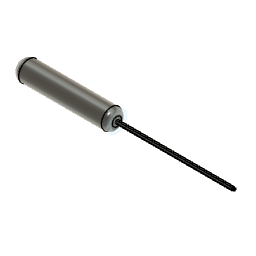
screwdriver v1 (Autodesk Fusion 360 design; units mm, degrees)
Autodesk Fusion 360 part; units mm, degrees
sketch "Sketch1" plane through (0, 0, 0) normal (1, 0, 0) x (0, 1, 0)
  circle A0 centre (0, 80) radius 13.595
  dimension "d2" = 27.19
  measures "d2" diameter of A0
extrude "Extrude1" add sketch "Sketch1" along normal blind 130
sketch "Sketch2" plane through (130, 0, 0) normal (1, 0, 0) x (0, 1, 0)
  circle A0 centre (0, 80) radius 13.595
  line L0 (1.1547, 78) -> (2.3094, 80)
  line L1 (2.3094, 80) -> (1.1547, 82)
  line L2 (1.1547, 82) -> (-1.1547, 82)
  line L3 (-1.1547, 82) -> (-2.3094, 80)
  line L4 (-2.3094, 80) -> (-1.1547, 78)
  line L5 (-1.1547, 78) -> (1.1547, 78)
  point P0 (0, 80)
  dimension "d5" = 2
  constraint coincident P0 A0.centre
  measures "d5" distance of P0 L5
extrude "Extrude2" add sketch "Sketch2" along normal blind 160 contours L0 L1 L2 L3 L4 L5
chamfer "Chamfer1" distance 1 angle 45 6 edges at (290, -1.7321, 81) (290, 0, 82) (290, -1.7321, 79) (290, 0, 78) (290, 1.7321, 79) (290, 1.7321, 81)
sketch "Sketch3" plane through (130, 0, 0) normal (1, 0, 0) x (0, 1, 0)
  line L0 (-1.1547, 78) -> (-2.3094, 80)
  line L1 (-2.3094, 80) -> (-1.1547, 82)
  line L2 (-1.1547, 82) -> (1.1547, 82)
  line L3 (1.1547, 82) -> (2.3094, 80)
  line L4 (2.3094, 80) -> (1.1547, 78)
  line L5 (1.1547, 78) -> (-1.1547, 78)
  circle A0 centre (0, 80) radius 13.595
sketch "Sketch4" plane through (290, 0, 0) normal (1, 0, 0) x (0, 1, 0)
  line L0 (0.5774, 79) -> (1.1547, 80)
  line L1 (1.1547, 80) -> (0.5774, 81)
  line L2 (0.5774, 81) -> (-0.5774, 81)
  line L3 (-0.5774, 81) -> (-1.1547, 80)
  line L4 (-1.1547, 80) -> (-0.5774, 79)
  line L5 (-0.5774, 79) -> (0.5774, 79)
  line L6 (-0.2, 80.1) -> (-0.2, 82.1)
  line L7 (-0.2, 82.1) -> (-2.8, 82.1)
  line L8 (-2.8, 82.1) -> (-2.8, 80.1)
  line L9 (-2.8, 80.1) -> (-0.2, 80.1)
  line L10 (0.2, 80.1) -> (0.2, 82.1)
  line L11 (0.2, 82.1) -> (2.8, 82.1)
  line L12 (2.8, 82.1) -> (2.8, 80.1)
  line L13 (2.8, 80.1) -> (0.2, 80.1)
  line L14 (0.2, 79.8) -> (2.8, 79.8)
  line L15 (2.8, 79.8) -> (2.8, 77.7841)
  line L16 (2.8, 77.7841) -> (0.2, 77.7841)
  line L17 (0.2, 77.7841) -> (0.2, 79.8)
  line L18 (-0.2, 79.8) -> (-0.2, 77.7841)
  line L19 (-0.2, 77.7841) -> (-2.5, 77.5)
  line L20 (-2.5, 77.5) -> (-2.5, 79.8)
  line L21 (-2.5, 79.8) -> (-0.2, 79.8)
  constraint perpendicular L2 L6
  constraint perpendicular L6 L7
  constraint perpendicular L7 L8
  constraint perpendicular L6 L9
  constraint perpendicular L9 L10
  constraint perpendicular L6 L11
  constraint perpendicular L11 L12
  constraint perpendicular L10 L13
  constraint perpendicular L10 L14
  constraint perpendicular L14 L15
  constraint perpendicular L10 L16
  constraint perpendicular L14 L17
  constraint perpendicular L5 L18
  constraint perpendicular L5 L20
  constraint perpendicular L18 L21
extrude "Extrude3" cut sketch "Sketch4" against normal blind 3 contours L0 L5 L14 L17 | L0 L5 L14 L15 L16 L17 | L4 L5 L18 L19 L20 L21 | L4 L5 L18 L21 | L1 L2 L10 L13 | L1 L2 L10 L11 L12 L13 | L2 L3 L6 L9 | L2 L3 L6 L7 L8 L9
fillet "Fillet1" radius 7.5 1 edges at (130, -12.675, 75.0838)
fillet "Fillet2" radius 10.5 1 edges at (0, -12.675, 75.0838)
equation "diamiter = 27.19 mm"
equation "d2 = diamiter"
